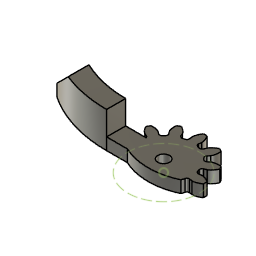
TRGRIP01_Grip_Left_50x15 (Autodesk Fusion 360 design; units mm, degrees)
description: Spur Gear; Module: 2.5; Num Teeth: 12; Pressure Angle: 20.0; Backlash: 0.00 mm
Autodesk Fusion 360 part; units mm, degrees
sketch "스케치1" plane through (0, 0, 0) normal (0, 0, 1) x (1, 0, 0) in component "Spur Gear (12 teeth)"
  circle A0 centre (0, 0) radius 11.9492
  circle A1 centre (0, 0) radius 2.5
sketch "스케치2" plane through (0, 0, 0) normal (0, 0, 1) x (1, 0, 0) in component "Spur Gear (12 teeth)"
  spline S0 degree 5 poles (13.9458, -2.0479) (13.9559, -2.0494) (13.9759, -2.052) (14.0061, -2.0549) (14.0465, -2.057) (14.0972, -2.0572) (14.1481, -2.0556) (14.199, -2.0528) (14.2501, -2.0495) (14.3011, -2.0457) (14.3522, -2.0415) (14.4034, -2.0367) (14.4546, -2.0311) (14.5058, -2.0247) (14.5571, -2.0173) (14.6084, -2.0091) (14.6597, -2.0003) (14.7111, -1.9908) (14.7624, -1.9808) (14.8137, -1.9703) (14.8651, -1.9594) (14.9164, -1.9479) (14.9678, -1.9358) (15.0191, -1.9232) (15.0705, -1.91) (15.1218, -1.8963) (15.1731, -1.882) (15.2244, -1.8673) (15.2757, -1.8521) (15.3269, -1.8365) (15.3781, -1.8204) (15.4293, -1.8038) (15.4805, -1.7868) (15.5316, -1.7693) (15.5827, -1.7513) (15.6338, -1.7329) (15.6848, -1.7141) (15.7358, -1.6948) (15.7868, -1.6751) (15.8377, -1.655) (15.8886, -1.6345) (15.9394, -1.6136) (15.9902, -1.5922) (16.0409, -1.5705) (16.0916, -1.5483) (16.1422, -1.5258) (16.1928, -1.5028) (16.2433, -1.4794) (16.2937, -1.4557) (16.3441, -1.4316) (16.3944, -1.4071) (16.4447, -1.3822) (16.4949, -1.3569) (16.545, -1.3313) (16.5951, -1.3053) (16.6451, -1.2789) (16.695, -1.2521) (16.7448, -1.225) (16.7946, -1.1975) (16.8443, -1.1697) (16.8939, -1.1415) (16.9435, -1.1129) (16.9929, -1.084) (17.0423, -1.0548) (17.0916, -1.0251) (17.1408, -0.9952) (17.1899, -0.9649) (17.239, -0.9343) (17.2879, -0.9033) (17.3368, -0.8719) (17.3856, -0.8403) (17.4245, -0.8147) (17.4537, -0.7953) (17.4731, -0.7824) (17.4828, -0.7759) knots 0 0 0 0 0 0 0.01428571 0.02857143 0.04285714 0.05714286 0.07142857 0.08571429 0.1 0.11428571 0.12857143 0.14285714 0.15714286 0.17142857 0.18571429 0.2 0.21428571 0.22857143 0.24285714 0.25714286 0.27142857 0.28571429 0.3 0.31428571 0.32857143 0.34285714 0.35714286 0.37142857 0.38571429 0.4 0.41428571 0.42857143 0.44285714 0.45714286 0.47142857 0.48571429 0.5 0.51428571 0.52857143 0.54285714 0.55714286 0.57142857 0.58571429 0.6 0.61428571 0.62857143 0.64285714 0.65714286 0.67142857 0.68571429 0.7 0.71428571 0.72857143 0.74285714 0.75714286 0.77142857 0.78571429 0.8 0.81428571 0.82857143 0.84285714 0.85714286 0.87142857 0.88571429 0.9 0.91428571 0.92857143 0.94285714 0.95714286 0.97142857 0.98571429 1 1 1 1 1 1
  spline S1 degree 5 poles (13.9458, 2.0479) (13.9559, 2.0494) (13.9759, 2.052) (14.0061, 2.0549) (14.0465, 2.057) (14.0972, 2.0572) (14.1481, 2.0556) (14.199, 2.0528) (14.2501, 2.0495) (14.3011, 2.0457) (14.3522, 2.0415) (14.4034, 2.0367) (14.4546, 2.0311) (14.5058, 2.0247) (14.5571, 2.0173) (14.6084, 2.0091) (14.6597, 2.0003) (14.7111, 1.9908) (14.7624, 1.9808) (14.8137, 1.9703) (14.8651, 1.9594) (14.9164, 1.9479) (14.9678, 1.9358) (15.0191, 1.9232) (15.0705, 1.91) (15.1218, 1.8963) (15.1731, 1.882) (15.2244, 1.8673) (15.2757, 1.8521) (15.3269, 1.8365) (15.3781, 1.8204) (15.4293, 1.8038) (15.4805, 1.7868) (15.5316, 1.7693) (15.5827, 1.7513) (15.6338, 1.7329) (15.6848, 1.7141) (15.7358, 1.6948) (15.7868, 1.6751) (15.8377, 1.655) (15.8886, 1.6345) (15.9394, 1.6136) (15.9902, 1.5922) (16.0409, 1.5705) (16.0916, 1.5483) (16.1422, 1.5258) (16.1928, 1.5028) (16.2433, 1.4794) (16.2937, 1.4557) (16.3441, 1.4316) (16.3944, 1.4071) (16.4447, 1.3822) (16.4949, 1.3569) (16.545, 1.3313) (16.5951, 1.3053) (16.6451, 1.2789) (16.695, 1.2521) (16.7448, 1.225) (16.7946, 1.1975) (16.8443, 1.1697) (16.8939, 1.1415) (16.9435, 1.1129) (16.9929, 1.084) (17.0423, 1.0548) (17.0916, 1.0251) (17.1408, 0.9952) (17.1899, 0.9649) (17.239, 0.9343) (17.2879, 0.9033) (17.3368, 0.8719) (17.3856, 0.8403) (17.4245, 0.8147) (17.4537, 0.7953) (17.4731, 0.7824) (17.4828, 0.7759) knots 0 0 0 0 0 0 0.01428571 0.02857143 0.04285714 0.05714286 0.07142857 0.08571429 0.1 0.11428571 0.12857143 0.14285714 0.15714286 0.17142857 0.18571429 0.2 0.21428571 0.22857143 0.24285714 0.25714286 0.27142857 0.28571429 0.3 0.31428571 0.32857143 0.34285714 0.35714286 0.37142857 0.38571429 0.4 0.41428571 0.42857143 0.44285714 0.45714286 0.47142857 0.48571429 0.5 0.51428571 0.52857143 0.54285714 0.55714286 0.57142857 0.58571429 0.6 0.61428571 0.62857143 0.64285714 0.65714286 0.67142857 0.68571429 0.7 0.71428571 0.72857143 0.74285714 0.75714286 0.77142857 0.78571429 0.8 0.81428571 0.82857143 0.84285714 0.85714286 0.87142857 0.88571429 0.9 0.91428571 0.92857143 0.94285714 0.95714286 0.97142857 0.98571429 1 1 1 1 1 1
  arc A0 (17.4828, -0.7759) -> (17.4828, 0.7759) centre (0, 0) ccw
  line L0 (11.8125, -1.7361) -> (13.9458, -2.0479)
  line L1 (11.8125, 1.7361) -> (13.9458, 2.0479)
  line L2 (11.8125, -1.7361) -> (11.8125, 1.7361)
  point P0 (14.1908, -2.0531)
  point P1 (14.4394, -2.0327)
  point P2 (14.6902, -1.9946)
  point P3 (14.9425, -1.9417)
  point P4 (15.196, -1.8754)
  point P5 (15.4504, -1.7967)
  point P6 (15.7053, -1.7063)
  point P7 (15.9604, -1.6047)
  point P8 (16.2156, -1.4922)
  point P9 (16.4704, -1.3692)
  point P10 (16.7248, -1.2358)
  point P11 (16.9785, -1.0924)
  point P12 (17.2312, -0.939)
  point P13 (14.1908, 2.0531)
  point P14 (14.4394, 2.0327)
  point P15 (14.6902, 1.9946)
  point P16 (14.9425, 1.9417)
  point P17 (15.196, 1.8754)
  point P18 (15.4504, 1.7967)
  point P19 (15.7053, 1.7063)
  point P20 (15.9604, 1.6047)
  point P21 (16.2156, 1.4922)
  point P22 (16.4704, 1.3692)
  point P23 (16.7248, 1.2358)
  point P24 (16.9785, 1.0924)
  point P25 (17.2312, 0.939)
sketch "스케치3" plane through (0, 0, 0) normal (0, 0, 1) x (1, 0, 0) in component "Spur Gear (12 teeth)"
sketch "스케치1 (2)" plane through (0, 0, 0) normal (0, 0, 1) x (1, 0, 0) in component "Spur Gear (12 teeth) (1)"
  circle A0 centre (0, 0) radius 11.9492
  circle A1 centre (0, 0) radius 2.5
  dimension "d44" = 5
  measures "d44" diameter of A1
extrude "돌출1" add sketch "스케치1 (2)" along normal blind 5 in component "Spur Gear (12 teeth) (1)"
sketch "스케치2 (2)" plane through (0, 0, 0) normal (0, 0, 1) x (1, 0, 0) in component "Spur Gear (12 teeth) (1)"
  spline S0 degree 5 poles (13.9458, -2.0479) (13.9559, -2.0494) (13.9759, -2.052) (14.0061, -2.0549) (14.0465, -2.057) (14.0972, -2.0572) (14.1481, -2.0556) (14.199, -2.0528) (14.2501, -2.0495) (14.3011, -2.0457) (14.3522, -2.0415) (14.4034, -2.0367) (14.4546, -2.0311) (14.5058, -2.0247) (14.5571, -2.0173) (14.6084, -2.0091) (14.6597, -2.0003) (14.7111, -1.9908) (14.7624, -1.9808) (14.8137, -1.9703) (14.8651, -1.9594) (14.9164, -1.9479) (14.9678, -1.9358) (15.0191, -1.9232) (15.0705, -1.91) (15.1218, -1.8963) (15.1731, -1.882) (15.2244, -1.8673) (15.2757, -1.8521) (15.3269, -1.8365) (15.3781, -1.8204) (15.4293, -1.8038) (15.4805, -1.7868) (15.5316, -1.7693) (15.5827, -1.7513) (15.6338, -1.7329) (15.6848, -1.7141) (15.7358, -1.6948) (15.7868, -1.6751) (15.8377, -1.655) (15.8886, -1.6345) (15.9394, -1.6136) (15.9902, -1.5922) (16.0409, -1.5705) (16.0916, -1.5483) (16.1422, -1.5258) (16.1928, -1.5028) (16.2433, -1.4794) (16.2937, -1.4557) (16.3441, -1.4316) (16.3944, -1.4071) (16.4447, -1.3822) (16.4949, -1.3569) (16.545, -1.3313) (16.5951, -1.3053) (16.6451, -1.2789) (16.695, -1.2521) (16.7448, -1.225) (16.7946, -1.1975) (16.8443, -1.1697) (16.8939, -1.1415) (16.9435, -1.1129) (16.9929, -1.084) (17.0423, -1.0548) (17.0916, -1.0251) (17.1408, -0.9952) (17.1899, -0.9649) (17.239, -0.9343) (17.2879, -0.9033) (17.3368, -0.8719) (17.3856, -0.8403) (17.4245, -0.8147) (17.4537, -0.7953) (17.4731, -0.7824) (17.4828, -0.7759) knots 0 0 0 0 0 0 0.01428571 0.02857143 0.04285714 0.05714286 0.07142857 0.08571429 0.1 0.11428571 0.12857143 0.14285714 0.15714286 0.17142857 0.18571429 0.2 0.21428571 0.22857143 0.24285714 0.25714286 0.27142857 0.28571429 0.3 0.31428571 0.32857143 0.34285714 0.35714286 0.37142857 0.38571429 0.4 0.41428571 0.42857143 0.44285714 0.45714286 0.47142857 0.48571429 0.5 0.51428571 0.52857143 0.54285714 0.55714286 0.57142857 0.58571429 0.6 0.61428571 0.62857143 0.64285714 0.65714286 0.67142857 0.68571429 0.7 0.71428571 0.72857143 0.74285714 0.75714286 0.77142857 0.78571429 0.8 0.81428571 0.82857143 0.84285714 0.85714286 0.87142857 0.88571429 0.9 0.91428571 0.92857143 0.94285714 0.95714286 0.97142857 0.98571429 1 1 1 1 1 1
  spline S1 degree 5 poles (13.9458, 2.0479) (13.9559, 2.0494) (13.9759, 2.052) (14.0061, 2.0549) (14.0465, 2.057) (14.0972, 2.0572) (14.1481, 2.0556) (14.199, 2.0528) (14.2501, 2.0495) (14.3011, 2.0457) (14.3522, 2.0415) (14.4034, 2.0367) (14.4546, 2.0311) (14.5058, 2.0247) (14.5571, 2.0173) (14.6084, 2.0091) (14.6597, 2.0003) (14.7111, 1.9908) (14.7624, 1.9808) (14.8137, 1.9703) (14.8651, 1.9594) (14.9164, 1.9479) (14.9678, 1.9358) (15.0191, 1.9232) (15.0705, 1.91) (15.1218, 1.8963) (15.1731, 1.882) (15.2244, 1.8673) (15.2757, 1.8521) (15.3269, 1.8365) (15.3781, 1.8204) (15.4293, 1.8038) (15.4805, 1.7868) (15.5316, 1.7693) (15.5827, 1.7513) (15.6338, 1.7329) (15.6848, 1.7141) (15.7358, 1.6948) (15.7868, 1.6751) (15.8377, 1.655) (15.8886, 1.6345) (15.9394, 1.6136) (15.9902, 1.5922) (16.0409, 1.5705) (16.0916, 1.5483) (16.1422, 1.5258) (16.1928, 1.5028) (16.2433, 1.4794) (16.2937, 1.4557) (16.3441, 1.4316) (16.3944, 1.4071) (16.4447, 1.3822) (16.4949, 1.3569) (16.545, 1.3313) (16.5951, 1.3053) (16.6451, 1.2789) (16.695, 1.2521) (16.7448, 1.225) (16.7946, 1.1975) (16.8443, 1.1697) (16.8939, 1.1415) (16.9435, 1.1129) (16.9929, 1.084) (17.0423, 1.0548) (17.0916, 1.0251) (17.1408, 0.9952) (17.1899, 0.9649) (17.239, 0.9343) (17.2879, 0.9033) (17.3368, 0.8719) (17.3856, 0.8403) (17.4245, 0.8147) (17.4537, 0.7953) (17.4731, 0.7824) (17.4828, 0.7759) knots 0 0 0 0 0 0 0.01428571 0.02857143 0.04285714 0.05714286 0.07142857 0.08571429 0.1 0.11428571 0.12857143 0.14285714 0.15714286 0.17142857 0.18571429 0.2 0.21428571 0.22857143 0.24285714 0.25714286 0.27142857 0.28571429 0.3 0.31428571 0.32857143 0.34285714 0.35714286 0.37142857 0.38571429 0.4 0.41428571 0.42857143 0.44285714 0.45714286 0.47142857 0.48571429 0.5 0.51428571 0.52857143 0.54285714 0.55714286 0.57142857 0.58571429 0.6 0.61428571 0.62857143 0.64285714 0.65714286 0.67142857 0.68571429 0.7 0.71428571 0.72857143 0.74285714 0.75714286 0.77142857 0.78571429 0.8 0.81428571 0.82857143 0.84285714 0.85714286 0.87142857 0.88571429 0.9 0.91428571 0.92857143 0.94285714 0.95714286 0.97142857 0.98571429 1 1 1 1 1 1
  arc A0 (17.4828, -0.7759) -> (17.4828, 0.7759) centre (0, 0) ccw
  line L0 (11.8125, -1.7361) -> (13.9458, -2.0479)
  line L1 (11.8125, 1.7361) -> (13.9458, 2.0479)
  line L2 (11.8125, -1.7361) -> (11.8125, 1.7361)
  point P0 (14.1908, -2.0531)
  point P1 (14.4394, -2.0327)
  point P2 (14.6902, -1.9946)
  point P3 (14.9425, -1.9417)
  point P4 (15.196, -1.8754)
  point P5 (15.4504, -1.7967)
  point P6 (15.7053, -1.7063)
  point P7 (15.9604, -1.6047)
  point P8 (16.2156, -1.4922)
  point P9 (16.4704, -1.3692)
  point P10 (16.7248, -1.2358)
  point P11 (16.9785, -1.0924)
  point P12 (17.2312, -0.939)
  point P13 (14.1908, 2.0531)
  point P14 (14.4394, 2.0327)
  point P15 (14.6902, 1.9946)
  point P16 (14.9425, 1.9417)
  point P17 (15.196, 1.8754)
  point P18 (15.4504, 1.7967)
  point P19 (15.7053, 1.7063)
  point P20 (15.9604, 1.6047)
  point P21 (16.2156, 1.4922)
  point P22 (16.4704, 1.3692)
  point P23 (16.7248, 1.2358)
  point P24 (16.9785, 1.0924)
  point P25 (17.2312, 0.939)
extrude "돌출2" add sketch "스케치2 (2)" along normal blind 5 in component "Spur Gear (12 teeth) (1)"
fillet "필렛1" radius 1 2 edges at (11.8222, -1.7375, 2.5) (11.8222, 1.7375, 2.5) in component "Spur Gear (12 teeth) (1)"
pattern_circular "C-패턴1" count 7 over 180 about axis through (0, 0, 0) along (0, 0, 1) of "돌출2", "필렛1" in component "Spur Gear (12 teeth) (1)"
sketch "스케치3 (2)" plane through (0, 0, 0) normal (0, 0, 1) x (1, 0, 0) in component "Spur Gear (12 teeth) (1)"
  circle A0 centre (0, 0) radius 15 construction
sketch "스케치1 (3)" plane through (0, 0, 0) normal (0, 0, 1) x (1, 0, 0)
  line L0 (-50, 4) -> (-10, 4)
  line L1 (-10, 4) -> (-10, -4)
  line L2 (-10, -4) -> (-50, -4)
  line L3 (-50, -4) -> (-50, 4)
  dimension "d25" = 8
  dimension "d26" = 40
  dimension "d27" = 4
  dimension "d28" = 50
  constraint horizontal L0
  constraint vertical L1
  constraint horizontal L2
  constraint vertical L3
  measures "d25" distance of L0.start L2.end
  measures "d26" distance of L1.end L2.end
  measures "d27" vertical distance of origin L0.start
  measures "d28" distance of origin L3
extrude "돌출3" add sketch "스케치1 (3)" along normal blind 15 in component "Spur Gear (12 teeth) (1)"
extrude "돌출7" cut 1 faces at (-10, 1.3333, 8.3333) along direction (-1, 0, 0) blind 10 in component "Spur Gear (12 teeth) (1)"
sketch "스케치4" plane through (0, 4, 0) normal (0, 1, 0) x (-1, 0, 0)
  line L0 (20, 15) -> (50, 15)
  line L1 (50, 15) -> (50, 0)
  line L2 (50, 0) -> (20, 0)
  line L3 (20, 0) -> (20, 15)
  point P0 (20, 15)
  point P1 (50, 0)
  constraint horizontal L0
  constraint vertical L1
  constraint horizontal L2
  constraint vertical L3
  constraint coincident P1 L1.end
  constraint coincident P0 L0.start
extrude "돌출8" add sketch "스케치4" along normal blind 6 in component "Spur Gear (12 teeth) (1)"
chamfer "챔퍼1" distance 10 angle 45 1 edges at (-50, 0, 15) in component "Spur Gear (12 teeth) (1)"
sketch "스케치3 (3)" plane through (0, 0, 5) normal (0, 0, 1) x (-1, 0, 0)
  arc A0 (11.2598, 4) -> (-11.6529, 2.6446) centre (0, 0) ccw
  arc A1 (11.2598, 4) -> (-11.6529, 2.6446) centre (0, 0) ccw
  circle A2 centre (0, -20) radius 26.5101
  dimension "d50" = 20
  constraint vertical A0.centre A2.centre
  constraint coincident A0.start A2
  measures "d50" distance of A0.centre A2.centre
extrude "돌출10" cut sketch "스케치3 (3)" against normal blind 5 contours A0 A1 A2 in component "Spur Gear (12 teeth) (1)"
sketch "스케치5" plane through (0, 0, 0) normal (0, 0, -1) x (1, 0, 0)
  line L0 (-20, -10) -> (-50, -10)
  line L1 (-50, -10) -> (-20, -10)
  circle A0 centre (-20, -50) radius 46
  circle A1 centre (-20, -50) radius 54
  line L2 (-20, -10) -> (-20, -4)
  line L3 (-20, -10) -> (-42.7156, -10)
  line L4 (-20, 4) -> (-50, 4)
  line L5 (-50, 4) -> (-50, -5.1001)
  point P0 (-50, -10)
  point P1 (-20, -10)
  point P2 (-20, -4)
  point P3 (-20, 4)
  dimension "d61" = 20
  dimension "d62" = 50
  constraint coincident A0 P2
  constraint concentric A0 A1
  constraint coincident A1 P3
  constraint coincident P1 L0.start
  constraint coincident P2 L2.end
  constraint coincident L0 L3.end
  constraint coincident A0 L3.end
  constraint perpendicular L2 L3
  constraint coincident P3 L4.start
  constraint tangent A1 L4
  constraint horizontal L4
  constraint coincident A1 L5.end
  constraint perpendicular L4 L5
  measures "d61" horizontal distance of origin A0.centre
  measures "d62" vertical distance of origin A0.centre
extrude "돌출13" cut sketch "스케치5" against normal blind 15 contours L0 L1 A0 L2 L3 | A1 L4 L5 picked at (-21.9743, -6.1276) in component "Spur Gear (12 teeth) (1)"
component "Spur Gear (12 teeth)" placed x (1, 0, 0) y (0, 1, 0) z (0, 0, 1) at (0, 0, 0)
component "Spur Gear (12 teeth) (1)" placed x (1, 0, 0) y (0, 1, 0) z (0, 0, 1) at (0, 0, 0)
